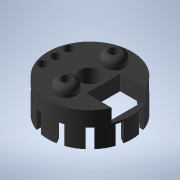
# Autodesk Inventor part: spacer
Saved by Autodesk Inventor 2020.2 (Build 242310000, 310)
## iProperties
Created: 2019-06-07
Part Number: spacer
Material: Generic
Document SubType Name: Modeling
Designer: Dammy
Density: 1 g/cm^3
Appearance: Default
Author: Dammy
Autodesk Inventor part; units mm, degrees
ref_plane "YZ Plane" through (0, 0, 0) normal (1, 0, 0) x (0, 1, 0)
ref_plane "XZ Plane" through (0, 0, 0) normal (0, 1, 0) x (-1, 0, 0)
ref_plane "XY Plane" through (0, 0, 0) normal (0, 0, 1) x (1, 0, 0)
sketch "Sketch1" plane through (0, 0, 0) normal (0, 1, 0) x (-1, 0, 0)
  circle A0 centre (0, 0) radius 22.25
  dimension "d0" = 44.5
  constraints: 1 centre point, 1 coincident
  measures "d0" diameter of A0
extrude "Extrusion1" add sketch "Sketch1" along normal blind 8
sketch "Sketch2" plane through (0, 8, 0) normal (0, 1, 0) x (1, 0, 0)
  circle A0 centre (0, 12.7) radius 2.6
  circle A1 centre (0, -12.7) radius 2.6
  point P0 (0, 0)
  dimension "d3" = 5.2
  dimension "d4" = 12.7
  dimension "d5" = 5.2
  dimension "d6" = 12.7
  constraints: 2 centre point, 2 vertical alignment
  measures "d3" diameter of A0
  measures "d4" distance of point (0, 0) A0.centre
  measures "d5" diameter of A1
  measures "d6" distance of point (0, 0) A1.centre
extrude "Extrusion2" cut sketch "Sketch2" against normal up to surface (8 mm away)
sketch "Sketch3" plane through (0, 8, 0) normal (0, 1, 0) x (1, 0, 0)
  circle A0 centre (0, 12.7) radius 2.6 projected
  circle A1 centre (0, 12.7) radius 2.6
  circle A2 centre (0, 12.7) radius 5.6
  point P0 (0, 0)
  dimension "d9" = 3
  constraints: 2 centre point, 2 coincident
  measures "d9" radial gap between concentric circles of A2 A0
extrude "Extrusion3" add sketch "Sketch3" along normal blind 5
mirror "Mirror1" about plane through (0, 0, 0) normal (0, 0, 1) of "Extrusion3"
sketch "Sketch4" plane through (0, 0, 0) normal (0, -1, 0) x (1, 0, 0)
  circle A0 centre (0, 0) radius 22.25 projected
  circle A1 centre (0, 0) radius 19.25
  circle A2 centre (0, 0) radius 22.25
  line L0 (2.5, -19.087) -> (-2.5, -19.087) construction
  line L1 (2.5, -19.087) -> (7.5, -19.087) construction
  line L2 (-2.5, -19.087) -> (-4.1056, -21.8679)
  line L3 (-2.5, -19.087) -> (0.7112, -19.087) construction
  line L4 (2.5, -19.087) -> (4.1056, -21.8679)
  line L5 (2.5, -19.087) -> (5.7112, -19.087) construction
  point P0 (4.1056, -21.8679)
  point P1 (-4.1056, -21.8679)
  dimension "d17" = 3
  dimension "d18" = 5
  dimension "d19" = 180
  dimension "d20" = 120
  dimension "d21" = 60
  constraints: 12 end point, 4 horizontal, 4 point on circle, 3 equal length, 2 centre point, 2 coincident, 1 concentric
  measures "d17" radial gap between concentric circles of A0 A1
  measures "d18" distance of L0.start L0.end
  measures "d19" angle of L0 L1
  measures "d20" angle of L2 L3
  measures "d21" angle of L4 L5
extrude "Extrusion5" add sketch "Sketch4" along normal blind 10 contours L2 A1 L4 A0 picked at (0.2785, -21.2156)
pattern_circular "Circular Pattern1" count 12 over 360 about axis through (0, -10, 0) along (0, 1, 0) of "Extrusion5"
fillet "Fillet1" radius 3 2 edges at (-5.6, 13, -12.7) (-5.6, 13, 12.7)
sketch "Sketch6" plane through (0, 8, 0) normal (0, 1, 0) x (1, 0, 0)
  circle A0 centre (0, 0) radius 22.25 projected
  circle A1 centre (0, 0) radius 22.25
  line L0 (7, 9) -> (7, -9)
  line L1 (7, 9) -> (25, 9) construction
  line L2 (7, 9) -> (20.3485, 9)
  line L3 (7, -9) -> (20.3485, -9)
  point P0 (7, 0)
  dimension "d29" = 18
  dimension "d30" = 90
  dimension "d56" = 7
  constraints: 8 end point, 2 horizontal, 2 point on circle, 1 centre point, 1 coincident, 1 concentric, 1 horizontal alignment, 1 midpoint, 1 perpendicular, 1 point on line, 1 vertical
  measures "d29" distance of L0.start L0.end
  measures "d30" angle of L0 L1
  measures "d56" distance from line of A0.centre L0
extrude "Extrusion6" cut sketch "Sketch6" against normal blind 7 contours A0 L3 L0 L2 picked at (12.0833, 0)
sketch "Sketch7" plane through (0, 8, 0) normal (0, 1, 0) x (1, 0, 0)
  circle A0 centre (0, 0) radius 19.25 construction
  arc A1 (20.3485, 9) -> (20.3485, -9) centre (0, 0) ccw construction
  circle A2 centre (3, 7) radius 2.5
  arc A3 (4.1056, 21.8679) -> (-4.1056, 21.8679) centre (0, 0) ccw construction
  line L0 (0, 22.25) -> (0, -22.25) construction
  arc A4 (-4.1056, -21.8679) -> (4.1056, -21.8679) centre (0, 0) ccw construction
  line L1 (22.25, 0) -> (-22.25, 0) construction
  arc A5 (-21.8679, 4.1056) -> (-21.8679, -4.1056) centre (0, 0) ccw construction
  line L2 (7, -9) -> (7, 9) construction
  circle A6 centre (3, 0) radius 2.5
  circle A7 centre (3, -7) radius 2.5
  circle A8 centre (0, 0) radius 5.5
  circle A9 centre (-18, 7) radius 2.5
  circle A10 centre (-18, 0) radius 2.5
  circle A11 centre (-18, -7) radius 2.5
  dimension "d51" = 10
  dimension "d34" = 3
  dimension "d35" = 5
  dimension "d36" = 4
  dimension "d39" = 7
  dimension "d44" = 11
  dimension "d45" = 5
  dimension "d48" = 7
  dimension "d53" = 21
  constraints: 8 centre point, 4 end point, 3 point on circle, 3 vertical, 2 coincident, 1 horizontal alignment, 1 midpoint, 1 perpendicular, 10 other
  measures "d35" diameter of A2
  measures "d36" distance from line of L2 A2.centre
  measures "d39" distance of A2.centre A6.centre
  measures "d44" diameter of A8
  measures "d45" diameter of A9
  measures "d48" distance of A9.centre A10.centre
  measures "d53" distance of A6.centre A10.centre
extrude "Extrusion7" cut sketch "Sketch7" against normal up to surface (8 mm away) contours A8 A2 | A6 | A2 A8 A7 | A7 A8 | A9 | A10 | A11 picked at (2.1127, 4.9296) picked at (2.1127, -4.9296)
sketch "Sketch9" plane through (0, 1, 0) normal (0, 1, 0) x (1, 0, 0)
  line L0 (7, -9) -> (7, 9) projected
  line L1 (20.3485, -9) -> (7, -9) projected
  line L2 (7, 9) -> (18.9991, 9)
  line L3 (18.9991, 9) -> (18.9991, -9)
  line L4 (18.9991, -9) -> (7, -9)
  line L5 (7, -9) -> (7, 9)
  point P0 (0, 0)
  constraints: 8 end point, 2 parallel, 1 horizontal, 1 perpendicular, 1 point on line
extrude "Extrusion8" cut sketch "Sketch9" against normal through all
equation "\"d5\" = d3"
equation "\"d6\" = d4"
equation "\"d34\" = d17"
equation "\"d45\" = d35"
body "Solid1"
